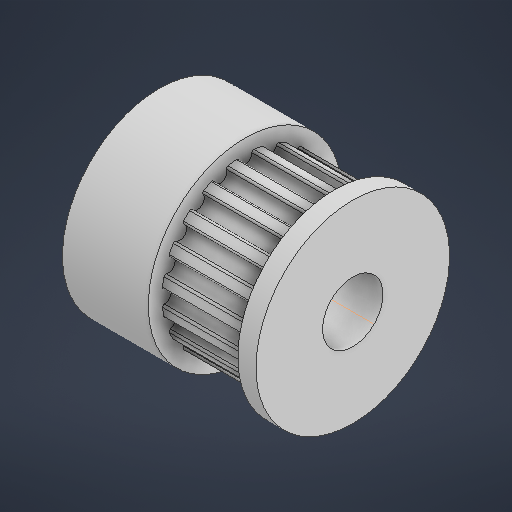
# Autodesk Inventor part: GT2Pulley_Tests
Saved by Autodesk Inventor 2025.2 (Build 292293000, 293)
## iProperties
Created: 2025-05-15
Part Number: GT2Pulley_Tests
Material: Generic
Document SubType Name: Modeling
Designer: Tiago
Density: 1 g/cm^3
Appearance: Default
Author: Tiago
Autodesk Inventor part; units mm, degrees
ref_plane "YZ Plane" through (0, 0, 0) normal (1, 0, 0) x (0, 1, 0)
ref_plane "XZ Plane" through (0, 0, 0) normal (0, 1, 0) x (-1, 0, 0)
ref_plane "XY Plane" through (0, 0, 0) normal (0, 0, 1) x (1, 0, 0)
sketch "Sketch1" plane through (0, 0, 0) normal (0, 0, 1) x (1, 0, 0)
  line L0 (0, 2.5) -> (0, 8.0002)
  line L1 (0, 8.0002) -> (7.1, 8.0002)
  line L2 (7.1, 8.0002) -> (7.1, 6.1102)
  line L3 (7.1, 6.1102) -> (14.5, 6.1102)
  line L4 (14.5, 6.1102) -> (14.5, 8.0002)
  line L5 (14.5, 8.0002) -> (16, 8.0002)
  line L6 (16, 8.0002) -> (16, 2.5)
  line L7 (16, 0) -> (0, 0)
  line L8 (0, 2.5) -> (16, 2.5)
  dimension "L" = 16
  dimension "d1" = 7.1
  dimension "DE" = 16.0004
  dimension "d3" = 12.2204
  dimension "d4" = 7.4
  dimension "d5" = 16.0004
  dimension "Bore" = 5
  constraints: 18 end point, 7 perpendicular, 2 vertical alignment, 1 horizontal, 1 vertical
  measures "L" distance of L7.start L7.end
  measures "d1" distance between parallel lines of L0 L2
  measures "DE" diameter of L1 L7
  measures "d3" diameter of L3 L7
  measures "d4" distance between parallel lines of L4 L2
  measures "d5" diameter of L5 L7
  measures "Bore" diameter of L8 L7
revolve "Revolution1" add sketch "Sketch1" angle 360 about axis through (16, 0, 0) along (-1, 0, 0)
sketch "Sketch3" plane through (7.1, 0, 0) normal (1, 0, 0) x (0, 0, -1)
  line L0 (0, 0) -> (0, 8.9731) construction
  line L1 (0, 0) -> (1.4779, 9.3313) construction
  line L2 (0, 0) -> (2.089, 9.3456) construction
  line L3 (0, 0) -> (2.8787, 8.8598) construction
  circle A0 centre (0, 0) radius 6.1102
  circle A1 centre (0, 0) radius 6.6652 construction
  arc A2 (1.5338, 6.5164) -> (1.4227, 6.711) centre (1.3916, 6.5643) ccw
  arc A3 (1.5338, 6.5164) -> (1.8882, 5.8111) centre (2.0597, 6.339) ccw
  arc A4 (0.7207, 6.8222) -> (0.555, 6.6714) centre (0.705, 6.6731) ccw
  arc A5 (0, 6.1102) -> (0.555, 6.6714) centre (0, 6.6652) ccw
  circle A6 centre (0, 0.0002) radius 6.3662 construction
  arc A7 (1.4227, 6.711) -> (0.7207, 6.8222) centre (0, 0) ccw
  point P0 (0, 6.1102)
  dimension "di" = 12.2204
  dimension "d12" = 0.555
  dimension "d8" = 9
  dimension "ANGLEP" = 18
  dimension "d10" = 3.6
  dimension "d16" = 0.3
  dimension "d17" = 0.555
  dimension "d18" = 0.15
  dimension "PD" = 12.7324
  constraints: 10 point on circle, 8 end point, 6 centre point, 5 symmetric about line, 2 tangent, 1 coincident, 1 point on line, 1 vertical, 8 other
  measures "d8" angle of L0 L1
  measures "ANGLEP" angle of L0 L3
  measures "d10" angle of L1 L2
  measures "d16" diameter of A2
  measures "d17" radius of A3
  measures "d18" radius of A2
  measures "PD" diameter of A6
extrude "Extrusion2" add sketch "Sketch3" along normal up to surface (7.4 mm away) contours A0 A5 A4 A7 A2 A3
pattern_circular "Circular Pattern2" count 20 over 360 about axis through (-10, 0, 0) along (1, 0, 0) of "Extrusion2"
equation "\"d3\" = di"
equation "\"d5\" = DE"
equation "\"d8\" = 0.5 * ANGLEP"
equation "\"d10\" = 0.2 * ANGLEP"
equation "\"PD\" = 0.63662 * zz"
equation "\"zz\" = 20"
body "Solid1"
